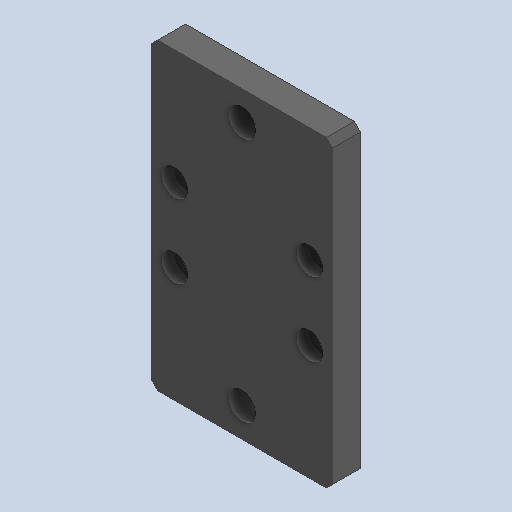
# Autodesk Inventor part: camera_mount
Saved by Autodesk Inventor 2024.2 (Build 282272000, 272)
## iProperties
Created: 2021-03-04
Part Number: camera_mount
Material: Generic
Document SubType Name: Modeling
Designer: maria
Density: 1 g/cm^3
Appearance: Default
Mass: 4.93692 g
Surface Area: 36.4997 cm^2
Volume: 4.93692 cm^3
Author: maria
Autodesk Inventor part; units mm, degrees
ref_plane "YZ Plane" through (0, 0, 0) normal (1, 0, 0) x (0, 1, 0)
ref_plane "XZ Plane" through (0, 0, 0) normal (0, 1, 0) x (-1, 0, 0)
ref_plane "XY Plane" through (0, 0, 0) normal (0, 0, 1) x (1, 0, 0)
sketch "Sketch1" plane through (0, 0, 0) normal (0, 0, 1) x (1, 0, 0)
  line L0 (-14.75, -15.25) -> (14.75, -15.25)
  line L1 (14.75, -15.25) -> (14.75, 15.25)
  line L2 (14.75, 15.25) -> (-14.75, 15.25)
  line L3 (-14.75, 15.25) -> (-14.75, -15.25)
  line L4 (-14.75, -15.25) -> (14.75, 15.25) construction
  line L5 (14.75, -15.25) -> (-14.75, 15.25) construction
  point P0 (0, 0)
  dimension "WIDTH" = 29.5
  dimension "LENGTH" = 30.5
  constraints: 12 end point, 2 midpoint, 2 parallel, 1 horizontal, 1 perpendicular
  measures "WIDTH" distance of L1.end L2.end
  measures "LENGTH" distance of L0.end L1.end
extrude "Extrusion1" add sketch "Sketch1" along normal blind 4.55
sketch "Sketch4" plane through (0, 0, 4.55) normal (0, 0, 1) x (1, 0, 0)
  line L0 (-14.75, 24.75) -> (14.75, 24.75)
  line L1 (14.75, 24.75) -> (14.75, -24.75)
  line L2 (14.75, -24.75) -> (-14.75, -24.75)
  line L3 (-14.75, -24.75) -> (-14.75, 24.75)
  line L4 (-14.75, 24.75) -> (14.75, -24.75) construction
  line L5 (14.75, 24.75) -> (-14.75, -24.75) construction
  point P0 (0, 0)
  dimension "LENGTH_WHOLE" = 49.5
  dimension "d30" = 29.5
  constraints: 12 end point, 2 midpoint, 2 parallel, 1 horizontal, 1 perpendicular
  measures "LENGTH_WHOLE" distance of L0.end L1.end
  measures "d30" distance of L1.end L2.end
extrude "Extrusion2" add sketch "Sketch4" against normal blind 4.55
sketch "Sketch2" plane through (0, 0, 4.55) normal (0, 0, 1) x (1, 0, 0)
  point P0 (0, 0)
  point P1 (-11, 6)
  point P2 (11, 6)
  point P3 (-11, -6)
  point P4 (11, -6)
  dimension "d11" = 22
  dimension "d12" = 0
  dimension "d13" = 0
  dimension "d14" = 0
  dimension "d15" = 0
  dimension "d16" = 12
  dimension "d17" = 6
  dimension "d18" = 11
  measures "d11" distance of point (11, 6) point (-11, 6)
  measures "d12" horizontal distance of point (-11, -6) point (-11, 6)
  measures "d13" vertical distance of point (11, 6) point (-11, 6)
  measures "d14" horizontal distance of point (11, -6) point (11, 6)
  measures "d15" vertical distance of point (-11, -6) point (11, -6)
  measures "d16" distance of point (11, -6) point (11, 6)
  measures "d17" vertical distance of point (11, 6) point (0, 0)
  measures "d18" horizontal distance of point (-11, -6) point (0, 0)
hole "Hole1" at (-11, 6, 4.55) at (11, 6, 4.55) at (-11, -6, 4.55) at (11, -6, 4.55) direction (0, 0, -1) diameter 2.4 end through all counterbore diameter 4.4 counterbore depth 2.1 clearance for "Socket Head Cap Screw" size "M2" standard "Ansi Metric M Profile"
sketch "Sketch5" plane through (0, 0, 0) normal (0, 0, -1) x (-1, 0, 0)
  point P0 (0, 0)
  point P1 (0, 20)
  point P2 (0, -20)
  dimension "d40" = 0
  dimension "d41" = 0
  dimension "d42" = 20
  dimension "d43" = 40
  measures "d40" horizontal distance of point (0, 0) point (0, 20)
  measures "d41" horizontal distance of point (0, 20) point (0, -20)
  measures "d42" distance of point (0, 0) point (0, 20)
  measures "d43" distance of point (0, -20) point (0, 20)
hole "Hole3" at (0, 20, 0) at (0, -20, 0) direction (0, 0, 1) diameter 4.5 end through all clearance for "Socket Head Cap Screw" size "#8" standard "Ansi Unified Screw Threads"
sketch "Sketch9" plane through (0, 0, 0) normal (0, 0, -1) x (-1, 0, 0)
  circle A0 centre (11, 6) radius 1.2 projected
  point P0 (0, 0)
  point P1 (11, -6)
  point P2 (-11, 6)
  point P3 (-11, -6)
  dimension "d79" = 0
  dimension "d80" = 0
  dimension "d81" = 0
  dimension "d82" = 12
  dimension "d83" = 0
  dimension "d84" = 22
  dimension "d85" = 0
  dimension "d86" = 0
  measures "d79" distance of A0.centre point (11, 6)
  measures "d80" distance of A0.centre point (11, 6)
  measures "d81" horizontal distance of point (11, -6) A0.centre
  measures "d82" distance of point (11, 6) point (11, -6)
  measures "d83" vertical distance of point (-11, 6) point (11, 6)
  measures "d84" distance of A0.centre point (-11, 6)
  measures "d85" vertical distance of point (-11, -6) point (11, -6)
  measures "d86" horizontal distance of point (-11, 6) point (-11, -6)
hole "Hole6" at (-11, 6, 0) at (-11, -6, 0) at (11, 6, 0) at (11, -6, 0) direction (0, 0, 1) diameter 3.75 depth 0.5
chamfer "Chamfer3" distance 1 angle 45 4 edges at (14.75, -24.75, 2.275) (-14.75, -24.75, 2.275) (-14.75, 24.75, 2.275) (14.75, 24.75, 2.275)
equation "\"d30\" = WIDTH"
equation "\"d43\" = 2 * d42"
body "Solid1"
